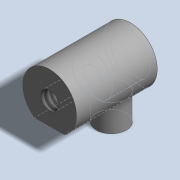
# Autodesk Inventor part: ShaftD6Female-632Female
Saved by Autodesk Inventor 2020 (Build 240168000, 168)
## iProperties
Created: 2021-07-07
Part Number: ShaftD6Female-632Female
Material: Generic
Document SubType Name: Modeling
Designer: Val
Density: 1 g/cm^3
Appearance: Default
Author: Val
Autodesk Inventor part; units mm, degrees
ref_plane "YZ Plane" through (0, 0, 0) normal (1, 0, 0) x (0, 1, 0)
ref_plane "XZ Plane" through (0, 0, 0) normal (0, 1, 0) x (-1, 0, 0)
ref_plane "XY Plane" through (0, 0, 0) normal (0, 0, 1) x (1, 0, 0)
sketch "Sketch1" plane through (0, 0, 0) normal (0, 0, 1) x (1, 0, 0)
  line L0 (-1.6583, -2.5) -> (1.6583, -2.5)
  arc A0 (1.6583, -2.5) -> (-1.6583, -2.5) centre (0, 0) ccw
  arc A1 (2.2111, -3.3333) -> (-2.2111, -3.3333) centre (0, 0) ccw
  line L1 (2.2111, -3.3333) -> (-2.2111, -3.3333)
  dimension "d0" = 1
  dimension "d1" = 3
  dimension "d2" = 3.3166
  dimension "d3" = 0.8333
  dimension "d4" = 3.3333
  dimension "d5" = 3.3333
  dimension "d6" = 4
  dimension "d7" = 0
  constraints: 4 end point, 4 point on circle, 2 centre point, 1 horizontal
  measures "d0" radial gap between concentric circles of A0 A1
  measures "d1" radius of A0
  measures "d2" distance of L0.start L0.end
  measures "d3" distance between parallel lines of L1 L0
  measures "d4" distance from line of point (0, 0) L1
  measures "d5" distance from line of point (0, 0) L1
  measures "d6" distance of point (0, 0) L1.start
  measures "d7" distance of point (0, 0) point (0, 0)
extrude "Extrusion1" add sketch "Sketch1" along normal blind 12
sketch "Sketch2" plane through (0, 0, 12) normal (0, 0, 1) x (1, 0, 0)
  arc A0 (2.2111, -3.3333) -> (-2.2111, -3.3333) centre (0, 0) ccw projected
  line L0 (-2.2111, -3.3333) -> (2.2111, -3.3333) projected
extrude "Extrusion2" add sketch "Sketch2" against normal blind 6.35
sketch "Sketch3" plane through (0, 0, 12) normal (0, 0, 1) x (1, 0, 0)
  point P0 (0, 0)
hole "Hole1" at (0, 0, 12) direction (0, 0, -1) diameter 2.6416 end through all thread size "6-32 UNC" class "2B" standard "ANSI Unified Screw Threads"
body "Solid1"
